# Autodesk Inventor part: switch
Saved by Autodesk Inventor 2013 (Build 170138000, 138)
## iProperties
Created: 2013-05-08
Part Number: switch
Material: Generic
Document SubType Name: Modeling
Designer: Administrator
Density: 1 g/cm^3
Author: Administrator
Autodesk Inventor part; units mm, degrees
ref_plane "YZ Plane" through (0, 0, 0) normal (1, 0, 0) x (0, 1, 0)
ref_plane "XZ Plane" through (0, 0, 0) normal (0, 1, 0) x (-1, 0, 0)
ref_plane "XY Plane" through (0, 0, 0) normal (0, 0, 1) x (1, 0, 0)
sketch "Sketch1" plane through (0, 0, 0) normal (0, 0, 1) x (1, 0, 0)
  line L0 (8.268, 4.6844) -> (8.268, -4.8156)
  line L1 (8.268, -4.8156) -> (-11.732, -4.8156)
  line L2 (-11.732, -4.8156) -> (-11.732, 5.3844)
  circle A0 centre (-6.482, -1.9156) radius 1.2
  circle A1 centre (3.018, -1.9156) radius 1.2
  line L3 (-9.425, 5.3844) -> (-9.425, 8.0844)
  line L4 (-9.425, 8.0844) -> (61.6567, 8.0844)
  line L5 (61.6567, 8.0844) -> (61.6567, 9.0844)
  line L6 (61.6567, 9.0844) -> (-10.3988, 9.0844)
  line L7 (-10.3988, 9.0844) -> (-10.3988, 5.3844)
  line L8 (-1.732, 5.3844) -> (-0.7437, 4.6844)
  line L9 (-0.7437, 4.6844) -> (8.268, 4.6844)
  line L10 (-11.732, 5.3844) -> (-10.3988, 5.3844)
  line L11 (-9.425, 5.3844) -> (-1.732, 5.3844)
  point P0 (0, 0)
  dimension "d0" = 20
  dimension "d2" = 2.4
  dimension "d3" = 2.4
  dimension "d4" = 9.5
  dimension "d5" = 5.25
  dimension "d6" = 2.9
  dimension "d7" = 2.9
  dimension "d8" = 10
  dimension "d9" = 11
  dimension "d10" = 9.5
  constraints: 24 end point, 6 parallel, 6 perpendicular, 2 centre point, 2 horizontal
  measures "d0" distance of L0.end L1.end
  measures "d2" diameter of A1
  measures "d3" diameter of A0
  measures "d4" distance of A0.centre A1.centre
  measures "d5" distance from line of L2 A0.centre
  measures "d6" distance from line of L1 A0.centre
  measures "d7" distance from line of L1 A1.centre
  measures "d8" distance from line of A1.centre L4
  measures "d9" distance from line of A1.centre L6
  measures "d10" distance between parallel lines of L1 L9
extrude "Extrusion1" add sketch "Sketch1" along normal blind 6.4
equation "\"d3\" = d2"
equation "\"d7\" = d6"
body "Solid1"
